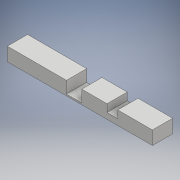
# Autodesk Inventor part: Cadru_2
Saved by Autodesk Inventor 2017 (Build 210142000, 142)
## iProperties
Created: 2017-06-13
Part Number: Cadru_2
Material: Generic
Document SubType Name: Modeling
Designer: crush
Density: 1 g/cm^3
Appearance: Default
Author: crush
Autodesk Inventor part; units mm, degrees
ref_plane "YZ Plane" through (0, 0, 0) normal (1, 0, 0) x (0, 1, 0)
ref_plane "XZ Plane" through (0, 0, 0) normal (0, 1, 0) x (-1, 0, 0)
ref_plane "XY Plane" through (0, 0, 0) normal (0, 0, 1) x (1, 0, 0)
sketch "Sketch1" plane through (0, 0, 0) normal (0, 1, 0) x (-1, 0, 0)
  line L0 (0, 0) -> (-430, 0)
  line L1 (-430, 0) -> (-430, -40)
  line L2 (-430, -40) -> (0, -40)
  line L3 (0, -40) -> (0, 0)
  dimension "d0" = 430
  dimension "d1" = 40
  constraints: 8 end point, 2 parallel, 1 horizontal, 1 perpendicular
  measures "d0" distance of L1.end L2.end
  measures "d1" distance of L2.end L0.start
extrude "Extrusion1" add sketch "Sketch1" along normal blind 60
sketch "Sketch2" plane through (0, 0, 0) normal (0, -1, 0) x (1, 0, 0)
  line L0 (430, 0) -> (430, -40)
  line L1 (430, -40) -> (0, -40)
  line L2 (361.5161, 0) -> (430, 0)
  line L3 (180.1999, -1.7586) -> (180.1999, -32.3586)
  line L4 (215.5999, -1.7586) -> (180.1999, -1.7586)
  line L5 (215.5999, -32.3586) -> (215.5999, -1.7586)
  line L6 (180.1999, -32.3586) -> (215.5999, -32.3586)
  line L7 (215.5999, -1.7586) -> (220.5999, -1.7586)
  line L8 (180.1999, -1.7586) -> (175.1999, -1.7586)
  line L9 (175.1999, -1.7586) -> (175.1999, 0)
  line L10 (430, -40) -> (0, -40) projected
  line L11 (220.5999, -1.7586) -> (220.5999, 0)
  line L12 (215.5999, -32.3586) -> (215.5999, -35.3586)
  line L13 (215.5999, -32.3586) -> (212.5999, -32.3586) construction
  line L14 (220.5999, 0) -> (175.1999, 0)
  line L15 (175.1999, 0) -> (175.1999, -35.3586)
  line L16 (175.1999, -35.3586) -> (220.5999, -35.3586)
  line L17 (220.5999, -35.3586) -> (220.5999, 0)
  point P0 (0, 0)
  point P1 (430, -40)
  dimension "d4" = 5
  dimension "d5" = 5
  dimension "d7" = 3
  dimension "d8" = 90
  constraints: 34 end point, 4 perpendicular, 2 parallel
  measures "d4" distance of L4.start L7.end
  measures "d5" distance of L3.start L8.end
  measures "d7" distance of L5.start L12.end
  measures "d8" angle of L13 L12
extrude "Extrusion2" cut sketch "Sketch2" against normal blind 60
sketch "Sketch4" plane through (0, 60, 0) normal (0, 1, 0) x (1, 0, 0)
  line L0 (220.5999, 0) -> (430, 0)
  line L1 (430, 40) -> (0, 40)
  line L2 (220.5999, 35.3586) -> (220.5999, 0)
  line L3 (175.1999, 0) -> (175.1999, 35.3586)
  line L4 (175.1999, 35.3586) -> (220.5999, 35.3586)
  line L5 (0, 0) -> (175.1999, 0)
  line L6 (300.8442, 17.7835) -> (300.8442, 2.5435)
  line L7 (321.1642, 2.5435) -> (321.1642, 17.7835)
  line L8 (300.8442, 2.5435) -> (321.1642, 2.5435)
  line L9 (321.1642, 17.7835) -> (300.8442, 17.7835)
  line L10 (220.5999, 0) -> (430, 0) projected
  line L11 (295.5283, 0) -> (327.2819, 0)
  line L12 (327.2819, 0) -> (327.2819, 22.353)
  line L13 (327.2819, 22.353) -> (295.5283, 22.353)
  line L14 (295.5283, 22.353) -> (295.5283, 0)
  constraints: 28 end point, 2 parallel, 1 horizontal, 1 perpendicular, 1 point on line
extrude "Extrusion3" cut sketch "Sketch4" against normal blind 60 contours L14 L13 L12 L0 | L9 L7 L8 L6
body "Solid1"
